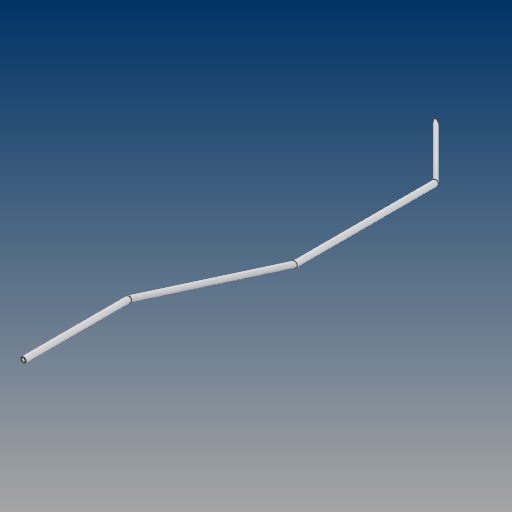
# Autodesk Inventor part: leg
Saved by Autodesk Inventor 2020 (Build 240168000, 168)
## iProperties
Created: 2020-09-14
Part Number: leg
Material: Generic
Document SubType Name: Modeling
Designer: alons
Density: 1 g/cm^3
Appearance: Default
Author: alons
Autodesk Inventor part; units mm, degrees
ref_plane "YZ Plane" through (0, 0, 0) normal (1, 0, 0) x (0, 1, 0)
ref_plane "XZ Plane" through (0, 0, 0) normal (0, 1, 0) x (-1, 0, 0)
ref_plane "XY Plane" through (0, 0, 0) normal (0, 0, 1) x (1, 0, 0)
sketch "Sketch1" plane through (0, 0, 0) normal (0, 1, 0) x (-1, 0, 0)
  line L0 (0, 0) -> (0, -10)
  line L1 (0, -10) -> (-5, -20.7225)
  line L2 (-5, -20.7225) -> (-5, -34.1134)
  line L3 (-5, -34.1134) -> (0, -39.1134)
  dimension "d0" = 10
  dimension "d1" = 5
  dimension "d2" = 155
  dimension "d3" = 135
  constraints: 8 end point, 1 parallel, 1 point on line, 1 vertical
  measures "d0" distance of L0.start L0.end
  measures "d1" distance from line of L2 L0.end
  measures "d2" angle of L2 L1
  measures "d3" angle of L3 L2
sketch "Sketch2" plane through (0, 0, 0) normal (0, 0, 1) x (1, 0, 0)
  circle A0 centre (0, 0) radius 0.25
  circle A1 centre (0, 0) radius 0.175
  dimension "d4" = 0.5
  dimension "d5" = 0.35
  constraints: 2 centre point, 2 coincident
  measures "d4" diameter of A0
  measures "d5" diameter of A1
sweep "Sweep1" add profiles "Sketch2" path "Sketch1" keep normal constant yes
body "Solid1"
